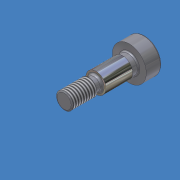
# Autodesk Inventor part: SCREW, SHOULDER, P, 12.9,  M6X10MM
Saved by Autodesk Inventor 2022.4 (Build 264492000, 492)
## iProperties
Created: 2001-02-28
Part Number: SCREW, SHOULDER, P, 12.9,  M6X10MM
Document SubType Name: Modeling
Designer: Peter Damgaard
Material: Steel, High Strength Low Alloy
Checked By: 1L5WN
Engr Approved By: P
User Status: Released
Description: SCREW, SHOULDER, P, 12.9,  M6X10MM
Mfg Approved By: Stephen.Oerton
Density: 7.84 g/cm^3
Appearance: Metal-Steel(Polish)
Mass: 6.19156 g
Surface Area: 6.6496 cm^2
Volume: 0.789739 cm^3
Company: Cooper Bussmann Denmark
Manager: 100-37122
Category: _
Shininess: 60.0
Density: 7.84
Volumn: 1.0724371659246204
Area: 8.535162991116971
PropertySet Name: Model Information
Control State: 0
Master: False
Checked Out: False
CN_SERVICEABLE: _
CN_MASS: 0.006192
CL_runCount: 1
FinishProperty: ToBeSet
FIRST_DESCRIPTION: SCREW, SHOULDER, P, 12.9,  M6X10MM
SECOND_DESCRIPTION: _
THIRD_DESCRIPTION: _
CN_DETAILER: -
CN_MFG_PART_NUM: _
CN_MFG_NAME: DEFAULT
STANDARDCLASSFLAG: P
CUSTOMERNUMBER: _
CN_DESIGNER: Stephen.Oerton
PTC_WM_ITERATION: 2
PTC_WM_ORGANIZATION_ID: CLWC
PTC_WM_LIFECYCLE: CLWC_CAD_LC
Title: SCREW, SHOULDER, P, 12_9,  M6X10MM_1L5WN.ipt
Author: -
Keywords: DEFAULT
Revision Number: 1
Subject: _
Autodesk Inventor part; units mm, degrees
ref_plane "YZ Plane" through (0, 0, 0) normal (1, 0, 0) x (0, 1, 0)
ref_plane "XZ Plane" through (0, 0, 0) normal (0, 1, 0) x (-1, 0, 0)
ref_plane "XY Plane" through (0, 0, 0) normal (0, 0, 1) x (1, 0, 0)
sketch "Sketch1" plane through (0, 0, 0) normal (0, 0, 1) x (1, 0, 0)
  line L0 (-4.5718, -2.6632) -> (-7.5718, -2.6632)
  line L1 (-7.5718, -2.6632) -> (-7.5718, -10.8132)
  line L2 (-7.5718, -10.8132) -> (-4.5718, -10.8132)
  line L3 (-4.5718, -10.8132) -> (-4.5718, -2.6632)
  dimension "d1" = 8.15
  dimension "d2" = 3
  constraints: 8 end point, 2 parallel, 1 perpendicular
  measures "d1" distance of L0.end L1.end
  measures "d2" distance of L0.start L0.end
revolve "Shoulder" add sketch "Sketch1" angle 360 about axis through (-4.5718, -10.8132, 0) along (0, 1, 0)
sketch "Sketch2" plane through (-4.5718, -2.6632, 0) normal (0, 1, 0) x (1, 0, 0)
  circle A0 centre (0, 0) radius 3 projected
  circle A1 centre (0, 0) radius 2.76
  dimension "d3" = 5.52
  constraints: 1 centre point, 1 concentric
  measures "d3" diameter of A1
extrude "Shoulder_neck" add sketch "Sketch2" along normal blind 1.85 contours A1
sketch "Sketch3" plane through (-4.5718, -0.8132, 0) normal (0, 1, 0) x (1, 0, 0)
  circle A0 centre (0, 0) radius 2.76 projected
  circle A1 centre (0, 0) radius 5.075
  dimension "d6" = 10.15
  constraints: 1 centre point, 1 concentric
  measures "d6" diameter of A1
extrude "Head" add sketch "Sketch3" along normal blind 4.5 contours A0 | A1
sketch "Sketch4" plane through (-4.5718, -10.8132, 0) normal (0, -1, 0) x (1, 0, 0)
  circle A0 centre (0, 0) radius 3 projected
  circle A1 centre (0, 0) radius 1.89
  dimension "d9" = 3.78
  constraints: 1 centre point, 1 concentric
  measures "d9" diameter of A1
extrude "Thread_neck" add sketch "Sketch4" along normal blind 1.8 contours A1
sketch "Sketch5" plane through (-4.5718, -12.6132, 0) normal (0, -1, 0) x (1, 0, 0)
  circle A0 centre (0, 0) radius 1.89 projected
  circle A1 centre (0, 0) radius 2.5
  dimension "d12" = 5
  constraints: 1 centre point, 1 concentric
  measures "d12" diameter of A1
extrude "Thread_shoulder" add sketch "Sketch5" along normal blind 7.7 contours A0 | A1
sketch "Sketch6" plane through (-4.5718, 3.6868, 0) normal (0, 1, 0) x (1, 0, 0)
  circle A0 centre (0, 0) radius 5.075 projected
  circle A1 centre (0, 0) radius 1.5 construction
  line L0 (-1.5, 0.866) -> (-1.5, -0.866)
  line L1 (-1.5, -0.866) -> (0, -1.7321)
  line L2 (0, -1.7321) -> (1.5, -0.866)
  line L3 (1.5, -0.866) -> (1.5, 0.866)
  line L4 (1.5, 0.866) -> (0, 1.7321)
  line L5 (0, 1.7321) -> (-1.5, 0.866)
  dimension "d15" = 3
  constraints: 12 end point, 6 equal length, 6 tangent, 1 centre point, 1 concentric, 1 parallel, 1 vertical
  measures "d15" diameter of A1
extrude "Hex" cut sketch "Sketch6" against normal blind 2.4 contours L5 L4 L3 L2 L1 L0
chamfer "Chamfer1" distance 0.24 angle 30 1 edges at (-1.5718, -2.6632, 0) measured on face at (-7.436, -2.6632, -0.4595)
fillet "Fillet1" radius 0.4 1 edges at (-7.3318, -0.8132, 0)
chamfer "Chamfer2" distance 0.3 angle 30 1 edges at (-9.6468, 3.6868, 0) measured on face at (0.4867, 2.1868, 0.4084)
chamfer "Chamfer3" distance 0.4 angle 30 1 edges at (-7.0718, -20.3132, 0) measured on face at (-3.3106, -20.3132, -0.6619)
fillet "Fillet2" radius 0.6 1 edges at (-6.4618, -10.8132, 0)
chamfer "Chamfer7" distance 0.61 angle 30 1 edges at (-7.0718, -12.6132, 0) measured on face at (-2.3177, -12.6132, -0.3502)
thread "Thread" size "M5x0.8" class "6g" standard "ANSI Metric M Profile" full length
equation "\"d1\" = Shoulder_length - Shoulder_neck_length"
equation "\"d2\" = 0.5 * Shoulder_diameter"
equation "\"d3\" = Shoulder_neck_dia"
equation "\"d4\" = Shoulder_neck_length"
equation "\"d6\" = Head_diameter"
equation "\"d7\" = Head_height"
equation "\"d9\" = Thread_neck_dia"
equation "\"d10\" = Thread_neck_length"
equation "\"d12\" = Thread_diameter"
equation "\"d13\" = Thread_length - Thread_neck_length"
equation "\"d15\" = Hex_size"
equation "\"d16\" = Hex_length"
equation "\"d18\" = -0.5 * Shoulder_neck_dia + 0.5 * Shoulder_diameter"
equation "\"d64\" = -0.5 * Shoulder_neck_dia + 0.5 * Shoulder_diameter"
equation "\"d21\" = 0.1 * Hex_size"
equation "\"d65\" = 0.1 * Hex_size"
equation "\"d23\" = 0.5 * Thread_pitch"
equation "\"d66\" = 0.5 * Thread_pitch"
equation "\"d25\" = Thread_neck_radius"
equation "\"d60\" = -0.5 * Thread_neck_dia + 0.5 * Thread_diameter"
equation "\"d67\" = -0.5 * Thread_neck_dia + 0.5 * Thread_diameter"
equation "\"Shoulder_diameter\" = 6"
equation "\"Shoulder_length\" = 10"
equation "\"Shoulder_neck_dia\" = 5.52"
equation "\"Thread_diameter\" = 5"
equation "\"Thread_length\" = 9.5"
equation "\"Head_diameter\" = 10.15"
equation "\"Head_height\" = 4.5"
equation "\"Thread_neck_dia\" = 3.78"
equation "\"Hex_size\" = 3"
equation "\"Hex_length\" = 2.4"
equation "\"Thread_pitch\" = 0.8"
equation "\"Shoulder_neck_length\" = 1.85"
equation "\"Thread_neck_length\" = 1.8"
equation "\"Thread_neck_radius\" = 0.6"
body "Solid1"
